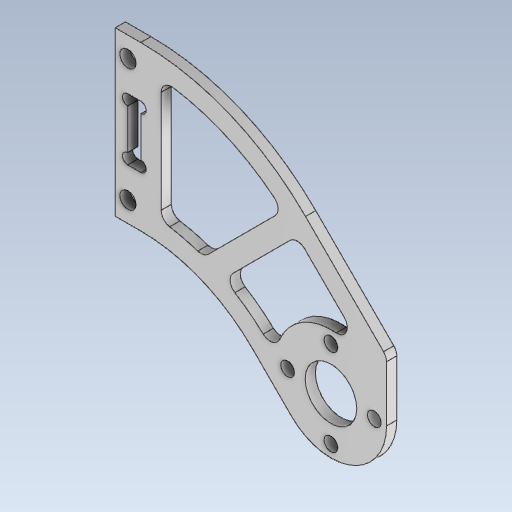
# Autodesk Inventor part: Shoulder_side_frame
Saved by Autodesk Inventor 2020.4 (Build 244396000, 396)
## iProperties
Created: 2022-01-10
Part Number: Shoulder_side_frame
Material: アルミニウム 2014-T4
Document SubType Name: Modeling
Designer: Masato Kubotera
Density: 2.8 g/cm^3
Appearance: 滑らか - 淡い灰色
Description: A2017 T2
Author: Masato Kubotera
Autodesk Inventor part; units mm, degrees
ref_plane "YZ Plane" through (0, 0, 0) normal (1, 0, 0) x (0, 1, 0)
ref_plane "XZ Plane" through (0, 0, 0) normal (0, 1, 0) x (-1, 0, 0)
ref_plane "XY Plane" through (0, 0, 0) normal (0, 0, 1) x (1, 0, 0)
sketch "スケッチ1" plane through (0, 0, 0) normal (1, 0, 0) x (0, 1, 0)
  line L0 (-42.3, 41) -> (-42.3, 9)
  line L1 (-42.3, 25) -> (-37.3, 25) construction
  line L2 (-39.8, 31) -> (-37.3, 31) construction
  line L3 (-37.3, 31) -> (-37.3, 19) construction
  line L4 (-37.3, 19) -> (-39.8, 19) construction
  line L5 (-39.8, 19) -> (-39.8, 31) construction
  line L6 (-39.8, 31) -> (-37.3, 19) construction
  line L7 (-37.3, 31) -> (-39.8, 19) construction
  circle A0 centre (-39.8, 37) radius 1.6
  line L8 (-39.8, 70.0011) -> (-39.8, -20.0011) construction
  line L9 (-42.3, 41) -> (-37.3, 41)
  circle A1 centre (0, 0) radius 5.05
  line L10 (0, 8.5) -> (0, -8.5) construction
  circle A2 centre (0, 8.5) radius 1.35
  arc A3 (-7.7075, -7.7075) -> (10.9, 0) centre (0, 0) ccw
  line L11 (-39.85, 31.05) -> (-37.25, 31.05)
  line L12 (-37.25, 31.05) -> (-37.25, 18.95)
  line L13 (-37.25, 18.95) -> (-39.85, 18.95)
  line L14 (-39.85, 18.95) -> (-39.85, 31.05)
  line L15 (-39.85, 31.05) -> (-37.25, 18.95) construction
  line L16 (-37.25, 31.05) -> (-39.85, 18.95) construction
  arc A4 (-37.25, 28.95) -> (-37.25, 31.05) centre (-37.25, 30) ccw
  line L17 (-38.55, 31) -> (-38.55, 19) construction
  arc A5 (-39.85, 31.05) -> (-39.85, 28.95) centre (-39.85, 30) ccw
  arc A6 (-37.25, 18.95) -> (-37.25, 21.05) centre (-37.25, 20) ccw
  arc A7 (-39.85, 21.05) -> (-39.85, 18.95) centre (-39.85, 20) ccw
  circle A8 centre (-39.8, 13) radius 1.6
  line L18 (-42.3, 9) -> (-37.3, 9)
  line L19 (-4.9889, 27.6163) -> (10.9, 11.7274)
  line L20 (10.9, 11.7274) -> (10.9, 0)
  line L21 (-15.3038, -0.1111) -> (-7.7075, -7.7075)
  circle A9 centre (-8.5, 0) radius 1.35
  circle A10 centre (0, -8.5) radius 1.35
  circle A11 centre (8.5, 0) radius 1.35
  circle A12 centre (0, 0) radius 16 construction
  arc A13 (-15.3038, -0.1111) -> (-37.3, 9) centre (-37.3, -22.1073) ccw
  line L22 (-37.3, 9) -> (-37.25, 9)
  arc A14 (-4.9889, 27.6163) -> (-37.3, 41) centre (-37.3, -4.6948) ccw
  line L23 (-33.3, 36.8077) -> (-33.3, 12.7714)
  arc A15 (-9.4163, 26.3045) -> (-33.3, 36.8077) centre (-37.3, -4.6948) ccw
  line L24 (-24.9607, 10.7601) -> (-9.4163, 26.3045)
  line L25 (-12.4754, 2.7173) -> (-10.8456, 1.0875)
  line L26 (-6.5912, 23.4727) -> (6.9, 9.9814)
  arc A16 (6.9, 8.438) -> (-10.8456, 1.0875) centre (0, 0) ccw
  line L27 (6.9, 9.9814) -> (6.9, 8.438)
  circle A17 centre (0, -8.5) radius 2.4 construction
  circle A18 centre (0, 8.5) radius 2.4 construction
  line L28 (-21.0507, 9.0132) -> (-6.5912, 23.4727)
  arc A19 (-12.4754, 2.7173) -> (-21.0507, 9.0132) centre (-37.3, -22.1073) ccw
  arc A20 (-24.9607, 10.7601) -> (-33.3, 12.7714) centre (-37.3, -22.1073) ccw
  point P0 (-38.55, 25)
  point P1 (-39.8, 25)
  point P2 (34.392, -0.1217)
  dimension "d0" = 5
  dimension "d1" = 32
  dimension "d2" = 2.5
  dimension "d3" = 12
  dimension "d4" = 3.2
  dimension "d5" = 5
  dimension "d6" = 10.1
  dimension "d7" = 17
  dimension "d8" = 2.7
  dimension "d10" = 42.3
  dimension "d11" = 1.05
  dimension "d12" = 0.05
  dimension "d13" = 0.05
  dimension "d14" = 24
  dimension "d15" = 25
  dimension "d19" = 360
  dimension "d23" = 32
  dimension "d24" = 45
  dimension "d26" = 4
  dimension "d29" = 4
  dimension "d31" = 4
  dimension "d32" = 4
  dimension "d36" = 4.8
  dimension "d37" = 4.8
  dimension "d39" = 4
  dimension "d40" = 4
  dimension "d41" = 1.797
  constraints: 56 end point, 22 point on circle, 21 centre point, 11 midpoint, 9 tangent, 8 coincident, 8 symmetric about line, 7 parallel, 5 point on line, 5 vertical, 4 horizontal, 3 perpendicular, 2 concentric, 17 other
  measures "d0" distance of L1.end L1.start
  measures "d1" distance of L0.start L0.end
  measures "d2" distance of L3.end L4.end
  measures "d3" distance of L2.end L3.end
  measures "d4" diameter of A0
  measures "d5" distance of L0.start A14.end
  measures "d6" diameter of A1
  measures "d7" distance of L10.start L10.end
  measures "d8" diameter of A2
  measures "d10" horizontal distance of A1.centre L0.end
  measures "d11" radius of A4
  measures "d12" distance between parallel lines of L2 L11
  measures "d13" distance between parallel lines of L3 L12
  measures "d14" distance of A8.centre A0.centre
  measures "d15" vertical distance of A1.centre L1.start
  measures "d23" diameter of A12
  measures "d24" angle of L0 L19
  measures "d26" radial gap between concentric circles of A15 A14
  measures "d29" distance between parallel lines of L21 L25
  measures "d31" distance between parallel lines of L20 L27
  measures "d32" distance between parallel lines of L23 L3
  measures "d36" diameter of A17
  measures "d37" diameter of A18
  measures "d39" radial gap between concentric circles of A13 A20
  measures "d40" distance between parallel lines of L28 L24
  measures "d41" distance from line of L19.start L28
extrude "押し出し1" add sketch "スケッチ1" along normal blind 2
fillet "フィレット1" radius 2 9 edges at (1, -33.3, 36.8077) (1, -10.8456, 1.0875) (1, 6.9, 8.438) (1, 6.9, 9.9814) (1, -33.3, 12.7714) (1, -24.9607, 10.7601) (1, -21.0507, 9.0132) (1, -6.5912, 23.4727) (1, -9.4163, 26.3045)
fillet "フィレット2" radius 2 1 edges at (1, 10.9, 11.7274)
equation "\"d13\" = d12"
